Autodesk Inventor part; units mm, degrees
(part 11 of 13)
  arc A3938 (16.5247, 22.3668) -> (16.5247, 22.5192) centre (16.5247, 22.443) ccw
  line L3943 (16.5247, 22.5192) -> (15.4062, 22.5192)
  arc A3939 (15.4062, 22.5192) -> (15.4062, 22.3668) centre (15.4062, 22.443) ccw
  line L3944 (16.6009, 22.0702) -> (16.6009, 22.8159)
  arc A3940 (16.6009, 22.8159) -> (16.4485, 22.8159) centre (16.5247, 22.8159) ccw
  line L3945 (16.4485, 22.8159) -> (16.4485, 22.0702)
  arc A3941 (16.4485, 22.0702) -> (16.6009, 22.0702) centre (16.5247, 22.0702) ccw
  line L3946 (15.4824, 23.2395) -> (15.4824, 23.6123)
  arc A3942 (15.4824, 23.6123) -> (15.33, 23.6123) centre (15.4062, 23.6123) ccw
  line L3947 (15.33, 23.6123) -> (15.33, 23.2395)
  arc A3943 (15.33, 23.2395) -> (15.4824, 23.2395) centre (15.4062, 23.2395) ccw
  line L3948 (15.4062, 23.3497) -> (16.5247, 23.3497)
  arc A3944 (16.5247, 23.3497) -> (16.5247, 23.5021) centre (16.5247, 23.4259) ccw
  line L3949 (16.5247, 23.5021) -> (15.4062, 23.5021)
  arc A3945 (15.4062, 23.5021) -> (15.4062, 23.3497) centre (15.4062, 23.4259) ccw
  line L3950 (16.6009, 23.2395) -> (16.6009, 23.6123)
  arc A3946 (16.6009, 23.6123) -> (16.4485, 23.6123) centre (16.5247, 23.6123) ccw
  line L3951 (16.4485, 23.6123) -> (16.4485, 23.2395)
  arc A3947 (16.4485, 23.2395) -> (16.6009, 23.2395) centre (16.5247, 23.2395) ccw
  line L3952 (16.4485, 24.5782) -> (16.4485, 24.2054)
  arc A3948 (16.4485, 24.2054) -> (16.6009, 24.2054) centre (16.5247, 24.2054) ccw
  line L3953 (16.6009, 24.2054) -> (16.6009, 24.5782)
  arc A3949 (16.6009, 24.5782) -> (16.4485, 24.5782) centre (16.5247, 24.5782) ccw
  line L3954 (16.4708, 24.2593) -> (16.2844, 24.0729)
  arc A3950 (16.2844, 24.0729) -> (16.3922, 23.9651) centre (16.3383, 24.019) ccw
  line L3955 (16.3922, 23.9651) -> (16.5786, 24.1515)
  arc A3951 (16.5786, 24.1515) -> (16.4708, 24.2593) centre (16.5247, 24.2054) ccw
  line L3956 (16.3383, 24.0952) -> (15.5926, 24.0952)
  arc A3952 (15.5926, 24.0952) -> (15.5926, 23.9428) centre (15.5926, 24.019) ccw
  line L3957 (15.5926, 23.9428) -> (16.3383, 23.9428)
  arc A3953 (16.3383, 23.9428) -> (16.3383, 24.0952) centre (16.3383, 24.019) ccw
  line L3958 (15.6465, 24.0729) -> (15.4601, 24.2593)
  arc A3954 (15.4601, 24.2593) -> (15.3523, 24.1515) centre (15.4062, 24.2054) ccw
  line L3959 (15.3523, 24.1515) -> (15.5387, 23.9651)
  arc A3955 (15.5387, 23.9651) -> (15.6465, 24.0729) centre (15.5926, 24.019) ccw
  line L3960 (15.4824, 24.2054) -> (15.4824, 24.5782)
  arc A3956 (15.4824, 24.5782) -> (15.33, 24.5782) centre (15.4062, 24.5782) ccw
  line L3961 (15.33, 24.5782) -> (15.33, 24.2054)
  arc A3957 (15.33, 24.2054) -> (15.4824, 24.2054) centre (15.4062, 24.2054) ccw
  line L3962 (15.4601, 24.5243) -> (15.6465, 24.7108)
  arc A3958 (15.6465, 24.7108) -> (15.5387, 24.8186) centre (15.5926, 24.7647) ccw
  line L3963 (15.5387, 24.8186) -> (15.3523, 24.6321)
  arc A3959 (15.3523, 24.6321) -> (15.4601, 24.5243) centre (15.4062, 24.5782) ccw
  line L3964 (15.5926, 24.6885) -> (16.3383, 24.6885)
  arc A3960 (16.3383, 24.6885) -> (16.3383, 24.8409) centre (16.3383, 24.7647) ccw
  line L3965 (16.3383, 24.8409) -> (15.5926, 24.8409)
  arc A3961 (15.5926, 24.8409) -> (15.5926, 24.6885) centre (15.5926, 24.7647) ccw
  line L3966 (16.2844, 24.7108) -> (16.4708, 24.5243)
  arc A3962 (16.4708, 24.5243) -> (16.5786, 24.6321) centre (16.5247, 24.5782) ccw
  line L3967 (16.5786, 24.6321) -> (16.3922, 24.8186)
  arc A3963 (16.3922, 24.8186) -> (16.2844, 24.7108) centre (16.3383, 24.7647) ccw
  line L3968 (15.4062, 25.1121) -> (16.5247, 25.1121)
  arc A3964 (16.5247, 25.1121) -> (16.5247, 25.2645) centre (16.5247, 25.1883) ccw
  line L3969 (16.5247, 25.2645) -> (15.4062, 25.2645)
  arc A3965 (15.4062, 25.2645) -> (15.4062, 25.1121) centre (15.4062, 25.1883) ccw
  line L3970 (16.567, 25.2517) -> (15.4485, 25.9974)
  arc A3966 (15.4485, 25.9974) -> (15.3639, 25.8706) centre (15.4062, 25.934) ccw
  line L3971 (15.3639, 25.8706) -> (16.4824, 25.1249)
  arc A3967 (16.4824, 25.1249) -> (16.567, 25.2517) centre (16.5247, 25.1883) ccw
  line L3972 (15.4062, 25.8578) -> (16.5247, 25.8578)
  arc A3968 (16.5247, 25.8578) -> (16.5247, 26.0102) centre (16.5247, 25.934) ccw
  line L3973 (16.5247, 26.0102) -> (15.4062, 26.0102)
  arc A3969 (15.4062, 26.0102) -> (15.4062, 25.8578) centre (15.4062, 25.934) ccw
  line L3974 (15.4062, 27.4507) -> (16.5247, 27.4507)
  arc A3970 (16.5247, 27.4507) -> (16.5247, 27.6031) centre (16.5247, 27.5269) ccw
  line L3975 (16.5247, 27.6031) -> (15.4062, 27.6031)
  arc A3971 (15.4062, 27.6031) -> (15.4062, 27.4507) centre (15.4062, 27.5269) ccw
  line L3976 (16.6009, 27.5269) -> (16.6009, 28.0861)
  arc A3972 (16.6009, 28.0861) -> (16.4485, 28.0861) centre (16.5247, 28.0861) ccw
  line L3977 (16.4485, 28.0861) -> (16.4485, 27.5269)
  arc A3973 (16.4485, 27.5269) -> (16.6009, 27.5269) centre (16.5247, 27.5269) ccw
  line L3978 (16.5786, 28.14) -> (16.3922, 28.3265)
  arc A3974 (16.3922, 28.3265) -> (16.2844, 28.2187) centre (16.3383, 28.2726) ccw
  line L3979 (16.2844, 28.2187) -> (16.4708, 28.0322)
  arc A3975 (16.4708, 28.0322) -> (16.5786, 28.14) centre (16.5247, 28.0861) ccw
  line L3980 (16.3383, 28.3488) -> (16.1519, 28.3488)
  arc A3976 (16.1519, 28.3488) -> (16.1519, 28.1964) centre (16.1519, 28.2726) ccw
  line L3981 (16.1519, 28.1964) -> (16.3383, 28.1964)
  arc A3977 (16.3383, 28.1964) -> (16.3383, 28.3488) centre (16.3383, 28.2726) ccw
  line L3982 (16.098, 28.3265) -> (15.9115, 28.14)
  arc A3978 (15.9115, 28.14) -> (16.0193, 28.0322) centre (15.9654, 28.0861) ccw
  line L3983 (16.0193, 28.0322) -> (16.2058, 28.2187)
  arc A3979 (16.2058, 28.2187) -> (16.098, 28.3265) centre (16.1519, 28.2726) ccw
  line L3984 (16.0193, 28.14) -> (15.8329, 28.3265)
  arc A3980 (15.8329, 28.3265) -> (15.7251, 28.2187) centre (15.779, 28.2726) ccw
  line L3985 (15.7251, 28.2187) -> (15.9115, 28.0322)
  arc A3981 (15.9115, 28.0322) -> (16.0193, 28.14) centre (15.9654, 28.0861) ccw
  line L3986 (15.779, 28.3488) -> (15.5926, 28.3488)
  arc A3982 (15.5926, 28.3488) -> (15.5926, 28.1964) centre (15.5926, 28.2726) ccw
  line L3987 (15.5926, 28.1964) -> (15.779, 28.1964)
  arc A3983 (15.779, 28.1964) -> (15.779, 28.3488) centre (15.779, 28.2726) ccw
  line L3988 (15.5387, 28.3265) -> (15.3523, 28.14)
  arc A3984 (15.3523, 28.14) -> (15.4601, 28.0322) centre (15.4062, 28.0861) ccw
  line L3989 (15.4601, 28.0322) -> (15.6465, 28.2187)
  arc A3985 (15.6465, 28.2187) -> (15.5387, 28.3265) centre (15.5926, 28.2726) ccw
  line L3990 (15.33, 28.0861) -> (15.33, 27.5269)
  arc A3986 (15.33, 27.5269) -> (15.4824, 27.5269) centre (15.4062, 27.5269) ccw
  line L3991 (15.4824, 27.5269) -> (15.4824, 28.0861)
  arc A3987 (15.4824, 28.0861) -> (15.33, 28.0861) centre (15.4062, 28.0861) ccw
  line L3992 (16.0416, 27.5269) -> (16.0416, 28.0861)
  arc A3988 (16.0416, 28.0861) -> (15.8892, 28.0861) centre (15.9654, 28.0861) ccw
  line L3993 (15.8892, 28.0861) -> (15.8892, 27.5269)
  arc A3989 (15.8892, 27.5269) -> (16.0416, 27.5269) centre (15.9654, 27.5269) ccw
  line L3994 (16.4485, 29.2554) -> (16.4485, 28.8826)
  arc A3990 (16.4485, 28.8826) -> (16.6009, 28.8826) centre (16.5247, 28.8826) ccw
  line L3995 (16.6009, 28.8826) -> (16.6009, 29.2554)
  arc A3991 (16.6009, 29.2554) -> (16.4485, 29.2554) centre (16.5247, 29.2554) ccw
  line L3996 (16.4708, 28.9365) -> (16.2844, 28.7501)
  arc A3992 (16.2844, 28.7501) -> (16.3922, 28.6423) centre (16.3383, 28.6962) ccw
  line L3997 (16.3922, 28.6423) -> (16.5786, 28.8287)
  arc A3993 (16.5786, 28.8287) -> (16.4708, 28.9365) centre (16.5247, 28.8826) ccw
  line L3998 (16.3383, 28.7724) -> (15.5926, 28.7724)
  arc A3994 (15.5926, 28.7724) -> (15.5926, 28.62) centre (15.5926, 28.6962) ccw
  line L3999 (15.5926, 28.62) -> (16.3383, 28.62)
  arc A3995 (16.3383, 28.62) -> (16.3383, 28.7724) centre (16.3383, 28.6962) ccw
  line L4000 (15.6465, 28.7501) -> (15.4601, 28.9365)
  arc A3996 (15.4601, 28.9365) -> (15.3523, 28.8287) centre (15.4062, 28.8826) ccw
  line L4001 (15.3523, 28.8287) -> (15.5387, 28.6423)
  arc A3997 (15.5387, 28.6423) -> (15.6465, 28.7501) centre (15.5926, 28.6962) ccw
  line L4002 (15.4824, 28.8826) -> (15.4824, 29.2554)
  arc A3998 (15.4824, 29.2554) -> (15.33, 29.2554) centre (15.4062, 29.2554) ccw
  line L4003 (15.33, 29.2554) -> (15.33, 28.8826)
  arc A3999 (15.33, 28.8826) -> (15.4824, 28.8826) centre (15.4062, 28.8826) ccw
  line L4004 (15.4601, 29.2015) -> (15.6465, 29.388)
  arc A4000 (15.6465, 29.388) -> (15.5387, 29.4958) centre (15.5926, 29.4419) ccw
  line L4005 (15.5387, 29.4958) -> (15.3523, 29.3093)
  arc A4001 (15.3523, 29.3093) -> (15.4601, 29.2015) centre (15.4062, 29.2554) ccw
  line L4006 (15.5926, 29.3657) -> (16.3383, 29.3657)
  arc A4002 (16.3383, 29.3657) -> (16.3383, 29.5181) centre (16.3383, 29.4419) ccw
  line L4007 (16.3383, 29.5181) -> (15.5926, 29.5181)
  arc A4003 (15.5926, 29.5181) -> (15.5926, 29.3657) centre (15.5926, 29.4419) ccw
  line L4008 (16.2844, 29.388) -> (16.4708, 29.2015)
  arc A4004 (16.4708, 29.2015) -> (16.5786, 29.3093) centre (16.5247, 29.2554) ccw
  line L4009 (16.5786, 29.3093) -> (16.3922, 29.4958)
  arc A4005 (16.3922, 29.4958) -> (16.2844, 29.388) centre (16.3383, 29.4419) ccw
  line L4010 (15.4062, 29.7893) -> (16.1519, 29.7893)
  arc A4006 (16.1519, 29.7893) -> (16.1519, 29.9417) centre (16.1519, 29.8655) ccw
  line L4011 (16.1519, 29.9417) -> (15.4062, 29.9417)
  arc A4007 (15.4062, 29.9417) -> (15.4062, 29.7893) centre (15.4062, 29.8655) ccw
  line L4012 (16.2058, 29.8116) -> (16.5786, 30.1844)
  arc A4008 (16.5786, 30.1844) -> (16.4708, 30.2922) centre (16.5247, 30.2383) ccw
  line L4013 (16.4708, 30.2922) -> (16.098, 29.9194)
  arc A4009 (16.098, 29.9194) -> (16.2058, 29.8116) centre (16.1519, 29.8655) ccw
  line L4014 (16.5786, 30.2922) -> (16.2058, 30.6651)
  arc A4010 (16.2058, 30.6651) -> (16.098, 30.5573) centre (16.1519, 30.6112) ccw
  line L4015 (16.098, 30.5573) -> (16.4708, 30.1844)
  arc A4011 (16.4708, 30.1844) -> (16.5786, 30.2922) centre (16.5247, 30.2383) ccw
  line L4016 (16.1519, 30.6874) -> (15.4062, 30.6874)
  arc A4012 (15.4062, 30.6874) -> (15.4062, 30.535) centre (15.4062, 30.6112) ccw
  line L4017 (15.4062, 30.535) -> (16.1519, 30.535)
  arc A4013 (16.1519, 30.535) -> (16.1519, 30.6874) centre (16.1519, 30.6112) ccw
  line L4018 (16.0416, 29.8655) -> (16.0416, 30.6112)
  arc A4014 (16.0416, 30.6112) -> (15.8892, 30.6112) centre (15.9654, 30.6112) ccw
  line L4019 (15.8892, 30.6112) -> (15.8892, 29.8655)
  arc A4015 (15.8892, 29.8655) -> (16.0416, 29.8655) centre (15.9654, 29.8655) ccw
  line L4020 (15.4062, 30.9586) -> (16.5247, 30.9586)
  arc A4016 (16.5247, 30.9586) -> (16.5247, 31.111) centre (16.5247, 31.0348) ccw
  line L4021 (16.5247, 31.111) -> (15.4062, 31.111)
  arc A4017 (15.4062, 31.111) -> (15.4062, 30.9586) centre (15.4062, 31.0348) ccw
  line L4022 (16.6009, 31.0348) -> (16.6009, 31.594)
  arc A4018 (16.6009, 31.594) -> (16.4485, 31.594) centre (16.5247, 31.594) ccw
  line L4023 (16.4485, 31.594) -> (16.4485, 31.0348)
  arc A4019 (16.4485, 31.0348) -> (16.6009, 31.0348) centre (16.5247, 31.0348) ccw
  line L4024 (16.5786, 31.6479) -> (16.3922, 31.8344)
  arc A4020 (16.3922, 31.8344) -> (16.2844, 31.7266) centre (16.3383, 31.7805) ccw
  line L4025 (16.2844, 31.7266) -> (16.4708, 31.5401)
  arc A4021 (16.4708, 31.5401) -> (16.5786, 31.6479) centre (16.5247, 31.594) ccw
  line L4026 (16.3383, 31.8567) -> (15.9654, 31.8567)
  arc A4022 (15.9654, 31.8567) -> (15.9654, 31.7043) centre (15.9654, 31.7805) ccw
  line L4027 (15.9654, 31.7043) -> (16.3383, 31.7043)
  arc A4023 (16.3383, 31.7043) -> (16.3383, 31.8567) centre (16.3383, 31.7805) ccw
  line L4028 (15.9115, 31.8344) -> (15.7251, 31.6479)
  arc A4024 (15.7251, 31.6479) -> (15.8329, 31.5401) centre (15.779, 31.594) ccw
  line L4029 (15.8329, 31.5401) -> (16.0193, 31.7266)
  arc A4025 (16.0193, 31.7266) -> (15.9115, 31.8344) centre (15.9654, 31.7805) ccw
  line L4030 (15.7028, 31.594) -> (15.7028, 31.0348)
  arc A4026 (15.7028, 31.0348) -> (15.8552, 31.0348) centre (15.779, 31.0348) ccw
  line L4031 (15.8552, 31.0348) -> (15.8552, 31.594)
  arc A4027 (15.8552, 31.594) -> (15.7028, 31.594) centre (15.779, 31.594) ccw
  line L4032 (15.8329, 31.4615) -> (15.4601, 31.8344)
  arc A4028 (15.4601, 31.8344) -> (15.3523, 31.7266) centre (15.4062, 31.7805) ccw
  line L4033 (15.3523, 31.7266) -> (15.7251, 31.3537)
  arc A4029 (15.7251, 31.3537) -> (15.8329, 31.4615) centre (15.779, 31.4076) ccw
  line L4034 (16.5247, 32.2803) -> (15.4062, 32.2803)
  arc A4030 (15.4062, 32.2803) -> (15.4062, 32.1279) centre (15.4062, 32.2041) ccw
  line L4035 (15.4062, 32.1279) -> (16.5247, 32.1279)
  arc A4031 (16.5247, 32.1279) -> (16.5247, 32.2803) centre (16.5247, 32.2041) ccw
  line L4036 (15.4824, 32.2041) -> (15.4824, 32.7633)
  arc A4032 (15.4824, 32.7633) -> (15.33, 32.7633) centre (15.4062, 32.7633) ccw
  line L4037 (15.33, 32.7633) -> (15.33, 32.2041)
  arc A4033 (15.33, 32.2041) -> (15.4824, 32.2041) centre (15.4062, 32.2041) ccw
  line L4038 (15.4601, 32.7094) -> (15.6465, 32.8959)
  arc A4034 (15.6465, 32.8959) -> (15.5387, 33.0037) centre (15.5926, 32.9498) ccw
  line L4039 (15.5387, 33.0037) -> (15.3523, 32.8172)
  arc A4035 (15.3523, 32.8172) -> (15.4601, 32.7094) centre (15.4062, 32.7633) ccw
  line L4040 (15.5926, 32.8736) -> (16.3383, 32.8736)
  arc A4036 (16.3383, 32.8736) -> (16.3383, 33.026) centre (16.3383, 32.9498) ccw
  line L4041 (16.3383, 33.026) -> (15.5926, 33.026)
  arc A4037 (15.5926, 33.026) -> (15.5926, 32.8736) centre (15.5926, 32.9498) ccw
  line L4042 (16.2844, 32.8959) -> (16.4708, 32.7094)
  arc A4038 (16.4708, 32.7094) -> (16.5786, 32.8172) centre (16.5247, 32.7633) ccw
  line L4043 (16.5786, 32.8172) -> (16.3922, 33.0037)
  arc A4039 (16.3922, 33.0037) -> (16.2844, 32.8959) centre (16.3383, 32.9498) ccw
  line L4044 (16.4485, 32.7633) -> (16.4485, 32.2041)
  arc A4040 (16.4485, 32.2041) -> (16.6009, 32.2041) centre (16.5247, 32.2041) ccw
  line L4045 (16.6009, 32.2041) -> (16.6009, 32.7633)
  arc A4041 (16.6009, 32.7633) -> (16.4485, 32.7633) centre (16.5247, 32.7633) ccw
  line L4046 (11.3544, 2.168) -> (11.5408, 1.9815)
  arc A4042 (11.5408, 1.9815) -> (11.6486, 2.0893) centre (11.5947, 2.0354) ccw
  line L4047 (11.6486, 2.0893) -> (11.4622, 2.2758)
  arc A4043 (11.4622, 2.2758) -> (11.3544, 2.168) centre (11.4083, 2.2219) ccw
  line L4048 (11.5185, 2.0354) -> (11.5185, 1.6626)
  arc A4044 (11.5185, 1.6626) -> (11.6709, 1.6626) centre (11.5947, 1.6626) ccw
  line L4049 (11.6709, 1.6626) -> (11.6709, 2.0354)
  arc A4045 (11.6709, 2.0354) -> (11.5185, 2.0354) centre (11.5947, 2.0354) ccw
  line L4050 (11.5408, 1.7165) -> (11.3544, 1.5301)
  arc A4046 (11.3544, 1.5301) -> (11.4622, 1.4223) centre (11.4083, 1.4762) ccw
  line L4051 (11.4622, 1.4223) -> (11.6486, 1.6087)
  arc A4047 (11.6486, 1.6087) -> (11.5408, 1.7165) centre (11.5947, 1.6626) ccw
  line L4052 (11.4083, 1.5524) -> (11.2219, 1.5524)
  arc A4048 (11.2219, 1.5524) -> (11.2219, 1.4) centre (11.2219, 1.4762) ccw
  line L4053 (11.2219, 1.4) -> (11.4083, 1.4)
  arc A4049 (11.4083, 1.4) -> (11.4083, 1.5524) centre (11.4083, 1.4762) ccw
  line L4054 (11.2758, 1.5301) -> (11.0893, 1.7165)
  arc A4050 (11.0893, 1.7165) -> (10.9815, 1.6087) centre (11.0354, 1.6626) ccw
  line L4055 (10.9815, 1.6087) -> (11.168, 1.4223)
  arc A4051 (11.168, 1.4223) -> (11.2758, 1.5301) centre (11.2219, 1.4762) ccw
  line L4056 (11.1116, 1.6626) -> (11.1116, 2.0354)
  arc A4052 (11.1116, 2.0354) -> (10.9592, 2.0354) centre (11.0354, 2.0354) ccw
  line L4057 (10.9592, 2.0354) -> (10.9592, 1.6626)
  arc A4053 (10.9592, 1.6626) -> (11.1116, 1.6626) centre (11.0354, 1.6626) ccw
  line L4058 (11.0893, 2.0893) -> (10.9029, 2.2758)
  arc A4054 (10.9029, 2.2758) -> (10.7951, 2.168) centre (10.849, 2.2219) ccw
  line L4059 (10.7951, 2.168) -> (10.9815, 1.9815)
  arc A4055 (10.9815, 1.9815) -> (11.0893, 2.0893) centre (11.0354, 2.0354) ccw
  line L4060 (10.849, 2.2981) -> (10.6626, 2.2981)
  arc A4056 (10.6626, 2.2981) -> (10.6626, 2.1457) centre (10.6626, 2.2219) ccw
  line L4061 (10.6626, 2.1457) -> (10.849, 2.1457)
  arc A4057 (10.849, 2.1457) -> (10.849, 2.2981) centre (10.849, 2.2219) ccw
  line L4062 (10.6087, 2.2758) -> (10.4223, 2.0893)
  arc A4058 (10.4223, 2.0893) -> (10.5301, 1.9815) centre (10.4762, 2.0354) ccw
  line L4063 (10.5301, 1.9815) -> (10.7165, 2.168)
  arc A4059 (10.7165, 2.168) -> (10.6087, 2.2758) centre (10.6626, 2.2219) ccw
  line L4064 (10.4, 2.0354) -> (10.4, 1.6626)
  arc A4060 (10.4, 1.6626) -> (10.5524, 1.6626) centre (10.4762, 1.6626) ccw
  line L4065 (10.5524, 1.6626) -> (10.5524, 2.0354)
  arc A4061 (10.5524, 2.0354) -> (10.4, 2.0354) centre (10.4762, 2.0354) ccw
  line L4066 (10.4223, 1.6087) -> (10.6087, 1.4223)
  arc A4062 (10.6087, 1.4223) -> (10.7165, 1.5301) centre (10.6626, 1.4762) ccw
  line L4067 (10.7165, 1.5301) -> (10.5301, 1.7165)
  arc A4063 (10.5301, 1.7165) -> (10.4223, 1.6087) centre (10.4762, 1.6626) ccw
  line L4068 (11.5185, 3.3912) -> (11.5185, 2.6455)
  arc A4064 (11.5185, 2.6455) -> (11.6709, 2.6455) centre (11.5947, 2.6455) ccw
  line L4069 (11.6709, 2.6455) -> (11.6709, 3.3912)
  arc A4065 (11.6709, 3.3912) -> (11.5185, 3.3912) centre (11.5947, 3.3912) ccw
  line L4070 (11.5947, 2.7217) -> (10.4762, 2.7217)
  arc A4066 (10.4762, 2.7217) -> (10.4762, 2.5693) centre (10.4762, 2.6455) ccw
  line L4071 (10.4762, 2.5693) -> (11.5947, 2.5693)
  arc A4067 (11.5947, 2.5693) -> (11.5947, 2.7217) centre (11.5947, 2.6455) ccw
  line L4072 (10.5524, 2.6455) -> (10.5524, 3.3912)
  arc A4068 (10.5524, 3.3912) -> (10.4, 3.3912) centre (10.4762, 3.3912) ccw
  line L4073 (10.4, 3.3912) -> (10.4, 2.6455)
  arc A4069 (10.4, 2.6455) -> (10.5524, 2.6455) centre (10.4762, 2.6455) ccw
  line L4074 (11.1116, 2.6455) -> (11.1116, 3.0183)
  arc A4070 (11.1116, 3.0183) -> (10.9592, 3.0183) centre (11.0354, 3.0183) ccw
  line L4075 (10.9592, 3.0183) -> (10.9592, 2.6455)
  arc A4071 (10.9592, 2.6455) -> (11.1116, 2.6455) centre (11.0354, 2.6455) ccw
  line L4076 (10.4762, 3.7386) -> (11.5947, 3.7386)
  arc A4072 (11.5947, 3.7386) -> (11.5947, 3.891) centre (11.5947, 3.8148) ccw
  line L4077 (11.5947, 3.891) -> (10.4762, 3.891)
  arc A4073 (10.4762, 3.891) -> (10.4762, 3.7386) centre (10.4762, 3.8148) ccw
  line L4078 (11.637, 3.8782) -> (10.5185, 4.6239)
  arc A4074 (10.5185, 4.6239) -> (10.4339, 4.4971) centre (10.4762, 4.5605) ccw
  line L4079 (10.4339, 4.4971) -> (11.5524, 3.7514)
  arc A4075 (11.5524, 3.7514) -> (11.637, 3.8782) centre (11.5947, 3.8148) ccw
  line L4080 (10.4762, 4.4843) -> (11.5947, 4.4843)
  arc A4076 (11.5947, 4.4843) -> (11.5947, 4.6367) centre (11.5947, 4.5605) ccw
  line L4081 (11.5947, 4.6367) -> (10.4762, 4.6367)
  arc A4077 (10.4762, 4.6367) -> (10.4762, 4.4843) centre (10.4762, 4.5605) ccw
  line L4082 (11.5947, 5.0603) -> (10.4762, 5.0603)
  arc A4078 (10.4762, 5.0603) -> (10.4762, 4.9079) centre (10.4762, 4.9841) ccw
  line L4083 (10.4762, 4.9079) -> (11.5947, 4.9079)
  arc A4079 (11.5947, 4.9079) -> (11.5947, 5.0603) centre (11.5947, 4.9841) ccw
  line L4084 (10.9029, 4.9302) -> (11.6486, 5.6759)
  arc A4080 (11.6486, 5.6759) -> (11.5408, 5.7837) centre (11.5947, 5.7298) ccw
  line L4085 (11.5408, 5.7837) -> (10.7951, 5.038)
  arc A4081 (10.7951, 5.038) -> (10.9029, 4.9302) centre (10.849, 4.9841) ccw
  line L4086 (11.0893, 5.2244) -> (10.5301, 5.7837)
  arc A4082 (10.5301, 5.7837) -> (10.4223, 5.6759) centre (10.4762, 5.7298) ccw
  line L4087 (10.4223, 5.6759) -> (10.9815, 5.1166)
  arc A4083 (10.9815, 5.1166) -> (11.0893, 5.2244) centre (11.0354, 5.1705) ccw
  line L4088 (11.5185, 6.7126) -> (11.5185, 6.3398)
  arc A4084 (11.5185, 6.3398) -> (11.6709, 6.3398) centre (11.5947, 6.3398) ccw
  line L4089 (11.6709, 6.3398) -> (11.6709, 6.7126)
  arc A4085 (11.6709, 6.7126) -> (11.5185, 6.7126) centre (11.5947, 6.7126) ccw
  line L4090 (11.5408, 6.3937) -> (11.3544, 6.2073)
  arc A4086 (11.3544, 6.2073) -> (11.4622, 6.0995) centre (11.4083, 6.1534) ccw
  line L4091 (11.4622, 6.0995) -> (11.6486, 6.2859)
  arc A4087 (11.6486, 6.2859) -> (11.5408, 6.3937) centre (11.5947, 6.3398) ccw
  line L4092 (11.4083, 6.2296) -> (10.6626, 6.2296)
  arc A4088 (10.6626, 6.2296) -> (10.6626, 6.0772) centre (10.6626, 6.1534) ccw
  line L4093 (10.6626, 6.0772) -> (11.4083, 6.0772)
  arc A4089 (11.4083, 6.0772) -> (11.4083, 6.2296) centre (11.4083, 6.1534) ccw
  line L4094 (10.7165, 6.2073) -> (10.5301, 6.3937)
  arc A4090 (10.5301, 6.3937) -> (10.4223, 6.2859) centre (10.4762, 6.3398) ccw
  line L4095 (10.4223, 6.2859) -> (10.6087, 6.0995)
  arc A4091 (10.6087, 6.0995) -> (10.7165, 6.2073) centre (10.6626, 6.1534) ccw
  line L4096 (10.5524, 6.3398) -> (10.5524, 6.7126)
  arc A4092 (10.5524, 6.7126) -> (10.4, 6.7126) centre (10.4762, 6.7126) ccw
  line L4097 (10.4, 6.7126) -> (10.4, 6.3398)
  arc A4093 (10.4, 6.3398) -> (10.5524, 6.3398) centre (10.4762, 6.3398) ccw
  line L4098 (10.5301, 6.6587) -> (10.7165, 6.8452)
  arc A4094 (10.7165, 6.8452) -> (10.6087, 6.953) centre (10.6626, 6.8991) ccw
  line L4099 (10.6087, 6.953) -> (10.4223, 6.7665)
  arc A4095 (10.4223, 6.7665) -> (10.5301, 6.6587) centre (10.4762, 6.7126) ccw
  line L4100 (10.6626, 6.8229) -> (11.4083, 6.8229)
  arc A4096 (11.4083, 6.8229) -> (11.4083, 6.9753) centre (11.4083, 6.8991) ccw
  line L4101 (11.4083, 6.9753) -> (10.6626, 6.9753)
  arc A4097 (10.6626, 6.9753) -> (10.6626, 6.8229) centre (10.6626, 6.8991) ccw
  line L4102 (11.3544, 6.8452) -> (11.5408, 6.6587)
  arc A4098 (11.5408, 6.6587) -> (11.6486, 6.7665) centre (11.5947, 6.7126) ccw
  line L4103 (11.6486, 6.7665) -> (11.4622, 6.953)
  arc A4099 (11.4622, 6.953) -> (11.3544, 6.8452) centre (11.4083, 6.8991) ccw
  line L4104 (11.5947, 8.5682) -> (10.4762, 8.5682)
  arc A4100 (10.4762, 8.5682) -> (10.4762, 8.4158) centre (10.4762, 8.492) ccw
  line L4105 (10.4762, 8.4158) -> (11.5947, 8.4158)
  arc A4101 (11.5947, 8.4158) -> (11.5947, 8.5682) centre (11.5947, 8.492) ccw
  line L4106 (10.5524, 8.492) -> (10.5524, 9.2377)
  arc A4102 (10.5524, 9.2377) -> (10.4, 9.2377) centre (10.4762, 9.2377) ccw
  line L4107 (10.4, 9.2377) -> (10.4, 8.492)
  arc A4103 (10.4, 8.492) -> (10.5524, 8.492) centre (10.4762, 8.492) ccw
  line L4108 (10.4762, 9.5851) -> (11.2219, 9.5851)
  arc A4104 (11.2219, 9.5851) -> (11.2219, 9.7375) centre (11.2219, 9.6613) ccw
  line L4109 (11.2219, 9.7375) -> (10.4762, 9.7375)
  arc A4105 (10.4762, 9.7375) -> (10.4762, 9.5851) centre (10.4762, 9.6613) ccw
  line L4110 (11.2758, 9.6074) -> (11.6486, 9.9802)
  arc A4106 (11.6486, 9.9802) -> (11.5408, 10.088) centre (11.5947, 10.0341) ccw
  line L4111 (11.5408, 10.088) -> (11.168, 9.7152)
  arc A4107 (11.168, 9.7152) -> (11.2758, 9.6074) centre (11.2219, 9.6613) ccw
  line L4112 (11.6486, 10.088) -> (11.2758, 10.4609)
  arc A4108 (11.2758, 10.4609) -> (11.168, 10.3531) centre (11.2219, 10.407) ccw
  line L4113 (11.168, 10.3531) -> (11.5408, 9.9802)
  arc A4109 (11.5408, 9.9802) -> (11.6486, 10.088) centre (11.5947, 10.0341) ccw
  line L4114 (11.2219, 10.4832) -> (10.4762, 10.4832)
  arc A4110 (10.4762, 10.4832) -> (10.4762, 10.3308) centre (10.4762, 10.407) ccw
  line L4115 (10.4762, 10.3308) -> (11.2219, 10.3308)
  arc A4111 (11.2219, 10.3308) -> (11.2219, 10.4832) centre (11.2219, 10.407) ccw
  line L4116 (11.1116, 9.6613) -> (11.1116, 10.407)
  arc A4112 (11.1116, 10.407) -> (10.9592, 10.407) centre (11.0354, 10.407) ccw
  line L4117 (10.9592, 10.407) -> (10.9592, 9.6613)
  arc A4113 (10.9592, 9.6613) -> (11.1116, 9.6613) centre (11.0354, 9.6613) ccw
  line L4118 (10.4762, 10.7544) -> (11.5947, 10.7544)
  arc A4114 (11.5947, 10.7544) -> (11.5947, 10.9068) centre (11.5947, 10.8306) ccw
  line L4119 (11.5947, 10.9068) -> (10.4762, 10.9068)
  arc A4115 (10.4762, 10.9068) -> (10.4762, 10.7544) centre (10.4762, 10.8306) ccw
  line L4120 (11.6709, 10.8306) -> (11.6709, 11.3898)
  arc A4116 (11.6709, 11.3898) -> (11.5185, 11.3898) centre (11.5947, 11.3898) ccw
  line L4121 (11.5185, 11.3898) -> (11.5185, 10.8306)
  arc A4117 (11.5185, 10.8306) -> (11.6709, 10.8306) centre (11.5947, 10.8306) ccw
  line L4122 (11.6486, 11.4437) -> (11.4622, 11.6302)
  arc A4118 (11.4622, 11.6302) -> (11.3544, 11.5224) centre (11.4083, 11.5763) ccw
  line L4123 (11.3544, 11.5224) -> (11.5408, 11.3359)
  arc A4119 (11.5408, 11.3359) -> (11.6486, 11.4437) centre (11.5947, 11.3898) ccw
  line L4124 (11.4083, 11.6525) -> (11.2219, 11.6525)
  arc A4120 (11.2219, 11.6525) -> (11.2219, 11.5001) centre (11.2219, 11.5763) ccw
  line L4125 (11.2219, 11.5001) -> (11.4083, 11.5001)
  arc A4121 (11.4083, 11.5001) -> (11.4083, 11.6525) centre (11.4083, 11.5763) ccw
  line L4126 (11.168, 11.6302) -> (10.9815, 11.4437)
  arc A4122 (10.9815, 11.4437) -> (11.0893, 11.3359) centre (11.0354, 11.3898) ccw
  line L4127 (11.0893, 11.3359) -> (11.2758, 11.5224)
  arc A4123 (11.2758, 11.5224) -> (11.168, 11.6302) centre (11.2219, 11.5763) ccw
  line L4128 (11.0893, 11.4437) -> (10.9029, 11.6302)
  arc A4124 (10.9029, 11.6302) -> (10.7951, 11.5224) centre (10.849, 11.5763) ccw
  line L4129 (10.7951, 11.5224) -> (10.9815, 11.3359)
  arc A4125 (10.9815, 11.3359) -> (11.0893, 11.4437) centre (11.0354, 11.3898) ccw
  line L4130 (10.849, 11.6525) -> (10.6626, 11.6525)
  arc A4126 (10.6626, 11.6525) -> (10.6626, 11.5001) centre (10.6626, 11.5763) ccw
  line L4131 (10.6626, 11.5001) -> (10.849, 11.5001)
  arc A4127 (10.849, 11.5001) -> (10.849, 11.6525) centre (10.849, 11.5763) ccw
  line L4132 (10.6087, 11.6302) -> (10.4223, 11.4437)
  arc A4128 (10.4223, 11.4437) -> (10.5301, 11.3359) centre (10.4762, 11.3898) ccw
  line L4133 (10.5301, 11.3359) -> (10.7165, 11.5224)
  arc A4129 (10.7165, 11.5224) -> (10.6087, 11.6302) centre (10.6626, 11.5763) ccw
  line L4134 (10.4, 11.3898) -> (10.4, 10.8306)
  arc A4130 (10.4, 10.8306) -> (10.5524, 10.8306) centre (10.4762, 10.8306) ccw
  line L4135 (10.5524, 10.8306) -> (10.5524, 11.3898)
  arc A4131 (10.5524, 11.3898) -> (10.4, 11.3898) centre (10.4762, 11.3898) ccw
  line L4136 (11.1116, 10.8306) -> (11.1116, 11.3898)
  arc A4132 (11.1116, 11.3898) -> (10.9592, 11.3898) centre (11.0354, 11.3898) ccw
  line L4137 (10.9592, 11.3898) -> (10.9592, 10.8306)
  arc A4133 (10.9592, 10.8306) -> (11.1116, 10.8306) centre (11.0354, 10.8306) ccw
  line L4138 (10.4762, 13.093) -> (11.5947, 13.093)
  arc A4134 (11.5947, 13.093) -> (11.5947, 13.2454) centre (11.5947, 13.1692) ccw
  line L4139 (11.5947, 13.2454) -> (10.4762, 13.2454)
  arc A4135 (10.4762, 13.2454) -> (10.4762, 13.093) centre (10.4762, 13.1692) ccw
  line L4140 (11.6709, 13.1692) -> (11.6709, 13.7284)
  arc A4136 (11.6709, 13.7284) -> (11.5185, 13.7284) centre (11.5947, 13.7284) ccw
  line L4141 (11.5185, 13.7284) -> (11.5185, 13.1692)
  arc A4137 (11.5185, 13.1692) -> (11.6709, 13.1692) centre (11.5947, 13.1692) ccw
  line L4142 (11.6486, 13.7823) -> (11.4622, 13.9688)
  arc A4138 (11.4622, 13.9688) -> (11.3544, 13.861) centre (11.4083, 13.9149) ccw
  line L4143 (11.3544, 13.861) -> (11.5408, 13.6745)
  arc A4139 (11.5408, 13.6745) -> (11.6486, 13.7823) centre (11.5947, 13.7284) ccw
  line L4144 (11.4083, 13.9911) -> (11.0354, 13.9911)
  arc A4140 (11.0354, 13.9911) -> (11.0354, 13.8387) centre (11.0354, 13.9149) ccw
  line L4145 (11.0354, 13.8387) -> (11.4083, 13.8387)
  arc A4141 (11.4083, 13.8387) -> (11.4083, 13.9911) centre (11.4083, 13.9149) ccw
  line L4146 (10.9815, 13.9688) -> (10.7951, 13.7823)
  arc A4142 (10.7951, 13.7823) -> (10.9029, 13.6745) centre (10.849, 13.7284) ccw
  line L4147 (10.9029, 13.6745) -> (11.0893, 13.861)
  arc A4143 (11.0893, 13.861) -> (10.9815, 13.9688) centre (11.0354, 13.9149) ccw
  line L4148 (10.7728, 13.7284) -> (10.7728, 13.1692)
  arc A4144 (10.7728, 13.1692) -> (10.9252, 13.1692) centre (10.849, 13.1692) ccw
  line L4149 (10.9252, 13.1692) -> (10.9252, 13.7284)
  arc A4145 (10.9252, 13.7284) -> (10.7728, 13.7284) centre (10.849, 13.7284) ccw
  line L4150 (11.5185, 14.8977) -> (11.5185, 14.5249)
  arc A4146 (11.5185, 14.5249) -> (11.6709, 14.5249) centre (11.5947, 14.5249) ccw
  line L4151 (11.6709, 14.5249) -> (11.6709, 14.8977)
  arc A4147 (11.6709, 14.8977) -> (11.5185, 14.8977) centre (11.5947, 14.8977) ccw
  line L4152 (11.5408, 14.5788) -> (11.3544, 14.3924)
  arc A4148 (11.3544, 14.3924) -> (11.4622, 14.2846) centre (11.4083, 14.3385) ccw
  line L4153 (11.4622, 14.2846) -> (11.6486, 14.471)
  arc A4149 (11.6486, 14.471) -> (11.5408, 14.5788) centre (11.5947, 14.5249) ccw
  line L4154 (11.4083, 14.4147) -> (10.6626, 14.4147)
  arc A4150 (10.6626, 14.4147) -> (10.6626, 14.2623) centre (10.6626, 14.3385) ccw
  line L4155 (10.6626, 14.2623) -> (11.4083, 14.2623)
  arc A4151 (11.4083, 14.2623) -> (11.4083, 14.4147) centre (11.4083, 14.3385) ccw
  line L4156 (10.7165, 14.3924) -> (10.5301, 14.5788)
  arc A4152 (10.5301, 14.5788) -> (10.4223, 14.471) centre (10.4762, 14.5249) ccw
  line L4157 (10.4223, 14.471) -> (10.6087, 14.2846)
  arc A4153 (10.6087, 14.2846) -> (10.7165, 14.3924) centre (10.6626, 14.3385) ccw
  line L4158 (10.5524, 14.5249) -> (10.5524, 14.8977)
  arc A4154 (10.5524, 14.8977) -> (10.4, 14.8977) centre (10.4762, 14.8977) ccw
  line L4159 (10.4, 14.8977) -> (10.4, 14.5249)
  arc A4155 (10.4, 14.5249) -> (10.5524, 14.5249) centre (10.4762, 14.5249) ccw
  line L4160 (10.5301, 14.8438) -> (10.7165, 15.0303)
  arc A4156 (10.7165, 15.0303) -> (10.6087, 15.1381) centre (10.6626, 15.0842) ccw
  line L4161 (10.6087, 15.1381) -> (10.4223, 14.9516)
  arc A4157 (10.4223, 14.9516) -> (10.5301, 14.8438) centre (10.4762, 14.8977) ccw
  line L4162 (10.6626, 15.008) -> (11.4083, 15.008)
  arc A4158 (11.4083, 15.008) -> (11.4083, 15.1604) centre (11.4083, 15.0842) ccw
  line L4163 (11.4083, 15.1604) -> (10.6626, 15.1604)
  arc A4159 (10.6626, 15.1604) -> (10.6626, 15.008) centre (10.6626, 15.0842) ccw
  line L4164 (11.3544, 15.0303) -> (11.5408, 14.8438)
  arc A4160 (11.5408, 14.8438) -> (11.6486, 14.9516) centre (11.5947, 14.8977) ccw
  line L4165 (11.6486, 14.9516) -> (11.4622, 15.1381)
  arc A4161 (11.4622, 15.1381) -> (11.3544, 15.0303) centre (11.4083, 15.0842) ccw
  line L4166 (11.5947, 15.584) -> (10.4762, 15.584)
  arc A4162 (10.4762, 15.584) -> (10.4762, 15.4316) centre (10.4762, 15.5078) ccw
  line L4167 (10.4762, 15.4316) -> (11.5947, 15.4316)
  arc A4163 (11.5947, 15.4316) -> (11.5947, 15.584) centre (11.5947, 15.5078) ccw
  line L4168 (10.5301, 15.4539) -> (10.9029, 15.8267)
  arc A4164 (10.9029, 15.8267) -> (10.7951, 15.9345) centre (10.849, 15.8806) ccw
  line L4169 (10.7951, 15.9345) -> (10.4223, 15.5617)
  arc A4165 (10.4223, 15.5617) -> (10.5301, 15.4539) centre (10.4762, 15.5078) ccw
  line L4170 (10.9029, 15.9345) -> (10.5301, 16.3074)
  arc A4166 (10.5301, 16.3074) -> (10.4223, 16.1996) centre (10.4762, 16.2535) ccw
  line L4171 (10.4223, 16.1996) -> (10.7951, 15.8267)
  arc A4167 (10.7951, 15.8267) -> (10.9029, 15.9345) centre (10.849, 15.8806) ccw
  line L4172 (10.4762, 16.1773) -> (11.5947, 16.1773)
  arc A4168 (11.5947, 16.1773) -> (11.5947, 16.3297) centre (11.5947, 16.2535) ccw
  line L4173 (11.5947, 16.3297) -> (10.4762, 16.3297)
  arc A4169 (10.4762, 16.3297) -> (10.4762, 16.1773) centre (10.4762, 16.2535) ccw
  line L4174 (11.5185, 17.4228) -> (11.5185, 16.6771)
  arc A4170 (11.5185, 16.6771) -> (11.6709, 16.6771) centre (11.5947, 16.6771) ccw
  line L4175 (11.6709, 16.6771) -> (11.6709, 17.4228)
  arc A4171 (11.6709, 17.4228) -> (11.5185, 17.4228) centre (11.5947, 17.4228) ccw
  line L4176 (11.5947, 16.7533) -> (10.4762, 16.7533)
  arc A4172 (10.4762, 16.7533) -> (10.4762, 16.6009) centre (10.4762, 16.6771) ccw
  line L4177 (10.4762, 16.6009) -> (11.5947, 16.6009)
  arc A4173 (11.5947, 16.6009) -> (11.5947, 16.7533) centre (11.5947, 16.6771) ccw
  line L4178 (10.5524, 16.6771) -> (10.5524, 17.4228)
  arc A4174 (10.5524, 17.4228) -> (10.4, 17.4228) centre (10.4762, 17.4228) ccw
  line L4179 (10.4, 17.4228) -> (10.4, 16.6771)
  arc A4175 (10.4, 16.6771) -> (10.5524, 16.6771) centre (10.4762, 16.6771) ccw
  line L4180 (11.1116, 16.6771) -> (11.1116, 17.0499)
  arc A4176 (11.1116, 17.0499) -> (10.9592, 17.0499) centre (11.0354, 17.0499) ccw
  line L4181 (10.9592, 17.0499) -> (10.9592, 16.6771)
  arc A4177 (10.9592, 16.6771) -> (11.1116, 16.6771) centre (11.0354, 16.6771) ccw
  line L4182 (10.4762, 17.7702) -> (11.5947, 17.7702)
  arc A4178 (11.5947, 17.7702) -> (11.5947, 17.9226) centre (11.5947, 17.8464) ccw
  line L4183 (11.5947, 17.9226) -> (10.4762, 17.9226)
  arc A4179 (10.4762, 17.9226) -> (10.4762, 17.7702) centre (10.4762, 17.8464) ccw
  line L4184 (11.6709, 17.8464) -> (11.6709, 18.4056)
  arc A4180 (11.6709, 18.4056) -> (11.5185, 18.4056) centre (11.5947, 18.4056) ccw
  line L4185 (11.5185, 18.4056) -> (11.5185, 17.8464)
  arc A4181 (11.5185, 17.8464) -> (11.6709, 17.8464) centre (11.5947, 17.8464) ccw
  line L4186 (11.6486, 18.4595) -> (11.4622, 18.646)
  arc A4182 (11.4622, 18.646) -> (11.3544, 18.5382) centre (11.4083, 18.5921) ccw
  line L4187 (11.3544, 18.5382) -> (11.5408, 18.3517)
  arc A4183 (11.5408, 18.3517) -> (11.6486, 18.4595) centre (11.5947, 18.4056) ccw
  line L4188 (11.4083, 18.6683) -> (11.0354, 18.6683)
  arc A4184 (11.0354, 18.6683) -> (11.0354, 18.5159) centre (11.0354, 18.5921) ccw
  line L4189 (11.0354, 18.5159) -> (11.4083, 18.5159)
  arc A4185 (11.4083, 18.5159) -> (11.4083, 18.6683) centre (11.4083, 18.5921) ccw
  line L4190 (10.9815, 18.646) -> (10.7951, 18.4595)
  arc A4186 (10.7951, 18.4595) -> (10.9029, 18.3517) centre (10.849, 18.4056) ccw
  line L4191 (10.9029, 18.3517) -> (11.0893, 18.5382)
  arc A4187 (11.0893, 18.5382) -> (10.9815, 18.646) centre (11.0354, 18.5921) ccw
  line L4192 (10.7728, 18.4056) -> (10.7728, 17.8464)
  arc A4188 (10.7728, 17.8464) -> (10.9252, 17.8464) centre (10.849, 17.8464) ccw
  line L4193 (10.9252, 17.8464) -> (10.9252, 18.4056)
  arc A4189 (10.9252, 18.4056) -> (10.7728, 18.4056) centre (10.849, 18.4056) ccw
  line L4194 (10.9029, 18.2731) -> (10.5301, 18.646)
  arc A4190 (10.5301, 18.646) -> (10.4223, 18.5382) centre (10.4762, 18.5921) ccw
  line L4195 (10.4223, 18.5382) -> (10.7951, 18.1653)
  arc A4191 (10.7951, 18.1653) -> (10.9029, 18.2731) centre (10.849, 18.2192) ccw
  line L4196 (11.5947, 20.2612) -> (10.4762, 20.2612)
  arc A4192 (10.4762, 20.2612) -> (10.4762, 20.1088) centre (10.4762, 20.185) ccw
  line L4197 (10.4762, 20.1088) -> (11.5947, 20.1088)
  arc A4193 (11.5947, 20.1088) -> (11.5947, 20.2612) centre (11.5947, 20.185) ccw
  line L4198 (10.5524, 20.185) -> (10.5524, 20.7442)
  arc A4194 (10.5524, 20.7442) -> (10.4, 20.7442) centre (10.4762, 20.7442) ccw
  line L4199 (10.4, 20.7442) -> (10.4, 20.185)
  arc A4195 (10.4, 20.185) -> (10.5524, 20.185) centre (10.4762, 20.185) ccw
  line L4200 (10.5301, 20.6903) -> (10.7165, 20.8768)
  arc A4196 (10.7165, 20.8768) -> (10.6087, 20.9846) centre (10.6626, 20.9307) ccw
  line L4201 (10.6087, 20.9846) -> (10.4223, 20.7981)
  arc A4197 (10.4223, 20.7981) -> (10.5301, 20.6903) centre (10.4762, 20.7442) ccw
  line L4202 (10.6626, 20.8545) -> (11.4083, 20.8545)
  arc A4198 (11.4083, 20.8545) -> (11.4083, 21.0069) centre (11.4083, 20.9307) ccw
  line L4203 (11.4083, 21.0069) -> (10.6626, 21.0069)
  arc A4199 (10.6626, 21.0069) -> (10.6626, 20.8545) centre (10.6626, 20.9307) ccw
  line L4204 (11.3544, 20.8768) -> (11.5408, 20.6903)
  arc A4200 (11.5408, 20.6903) -> (11.6486, 20.7981) centre (11.5947, 20.7442) ccw
  line L4205 (11.6486, 20.7981) -> (11.4622, 20.9846)
  arc A4201 (11.4622, 20.9846) -> (11.3544, 20.8768) centre (11.4083, 20.9307) ccw
  line L4206 (11.5185, 20.7442) -> (11.5185, 20.185)
  arc A4202 (11.5185, 20.185) -> (11.6709, 20.185) centre (11.5947, 20.185) ccw
  line L4207 (11.6709, 20.185) -> (11.6709, 20.7442)
  arc A4203 (11.6709, 20.7442) -> (11.5185, 20.7442) centre (11.5947, 20.7442) ccw
  line L4208 (10.5524, 21.3543) -> (10.5524, 21.7271)
  arc A4204 (10.5524, 21.7271) -> (10.4, 21.7271) centre (10.4762, 21.7271) ccw
  line L4209 (10.4, 21.7271) -> (10.4, 21.3543)
  arc A4205 (10.4, 21.3543) -> (10.5524, 21.3543) centre (10.4762, 21.3543) ccw
  line L4210 (10.4762, 21.4645) -> (11.5947, 21.4645)
  arc A4206 (11.5947, 21.4645) -> (11.5947, 21.6169) centre (11.5947, 21.5407) ccw
  line L4211 (11.5947, 21.6169) -> (10.4762, 21.6169)
  arc A4207 (10.4762, 21.6169) -> (10.4762, 21.4645) centre (10.4762, 21.5407) ccw
  line L4212 (11.6709, 21.3543) -> (11.6709, 21.7271)
  arc A4208 (11.6709, 21.7271) -> (11.5185, 21.7271) centre (11.5947, 21.7271) ccw
  line L4213 (11.5185, 21.7271) -> (11.5185, 21.3543)
  arc A4209 (11.5185, 21.3543) -> (11.6709, 21.3543) centre (11.5947, 21.3543) ccw
  line L4214 (11.3544, 22.8256) -> (11.5408, 22.6391)
  arc A4210 (11.5408, 22.6391) -> (11.6486, 22.7469) centre (11.5947, 22.693) ccw
  line L4215 (11.6486, 22.7469) -> (11.4622, 22.9334)
  arc A4211 (11.4622, 22.9334) -> (11.3544, 22.8256) centre (11.4083, 22.8795) ccw
  line L4216 (11.5185, 22.693) -> (11.5185, 22.3202)
  arc A4212 (11.5185, 22.3202) -> (11.6709, 22.3202) centre (11.5947, 22.3202) ccw
  line L4217 (11.6709, 22.3202) -> (11.6709, 22.693)
  arc A4213 (11.6709, 22.693) -> (11.5185, 22.693) centre (11.5947, 22.693) ccw
  line L4218 (11.5408, 22.3741) -> (11.3544, 22.1877)
  arc A4214 (11.3544, 22.1877) -> (11.4622, 22.0799) centre (11.4083, 22.1338) ccw
  line L4219 (11.4622, 22.0799) -> (11.6486, 22.2663)
  arc A4215 (11.6486, 22.2663) -> (11.5408, 22.3741) centre (11.5947, 22.3202) ccw
  line L4220 (11.4083, 22.21) -> (11.2219, 22.21)
  arc A4216 (11.2219, 22.21) -> (11.2219, 22.0576) centre (11.2219, 22.1338) ccw
  line L4221 (11.2219, 22.0576) -> (11.4083, 22.0576)
  arc A4217 (11.4083, 22.0576) -> (11.4083, 22.21) centre (11.4083, 22.1338) ccw
  line L4222 (11.2758, 22.1877) -> (11.0893, 22.3741)
  arc A4218 (11.0893, 22.3741) -> (10.9815, 22.2663) centre (11.0354, 22.3202) ccw
  line L4223 (10.9815, 22.2663) -> (11.168, 22.0799)
  arc A4219 (11.168, 22.0799) -> (11.2758, 22.1877) centre (11.2219, 22.1338) ccw
  line L4224 (11.1116, 22.3202) -> (11.1116, 22.693)
  arc A4220 (11.1116, 22.693) -> (10.9592, 22.693) centre (11.0354, 22.693) ccw
  line L4225 (10.9592, 22.693) -> (10.9592, 22.3202)
  arc A4221 (10.9592, 22.3202) -> (11.1116, 22.3202) centre (11.0354, 22.3202) ccw
  line L4226 (11.0893, 22.7469) -> (10.9029, 22.9334)
  arc A4222 (10.9029, 22.9334) -> (10.7951, 22.8256) centre (10.849, 22.8795) ccw
  line L4227 (10.7951, 22.8256) -> (10.9815, 22.6391)
  arc A4223 (10.9815, 22.6391) -> (11.0893, 22.7469) centre (11.0354, 22.693) ccw
  line L4228 (10.849, 22.9557) -> (10.6626, 22.9557)
  arc A4224 (10.6626, 22.9557) -> (10.6626, 22.8033) centre (10.6626, 22.8795) ccw
  line L4229 (10.6626, 22.8033) -> (10.849, 22.8033)
  arc A4225 (10.849, 22.8033) -> (10.849, 22.9557) centre (10.849, 22.8795) ccw
  line L4230 (10.6087, 22.9334) -> (10.4223, 22.7469)
  arc A4226 (10.4223, 22.7469) -> (10.5301, 22.6391) centre (10.4762, 22.693) ccw
  line L4231 (10.5301, 22.6391) -> (10.7165, 22.8256)
  arc A4227 (10.7165, 22.8256) -> (10.6087, 22.9334) centre (10.6626, 22.8795) ccw
  line L4232 (10.4, 22.693) -> (10.4, 22.3202)
  arc A4228 (10.4, 22.3202) -> (10.5524, 22.3202) centre (10.4762, 22.3202) ccw
  line L4233 (10.5524, 22.3202) -> (10.5524, 22.693)
  arc A4229 (10.5524, 22.693) -> (10.4, 22.693) centre (10.4762, 22.693) ccw
  line L4234 (10.4223, 22.2663) -> (10.6087, 22.0799)
  arc A4230 (10.6087, 22.0799) -> (10.7165, 22.1877) centre (10.6626, 22.1338) ccw
  line L4235 (10.7165, 22.1877) -> (10.5301, 22.3741)
  arc A4231 (10.5301, 22.3741) -> (10.4223, 22.2663) centre (10.4762, 22.3202) ccw
  line L4236 (10.4762, 23.5997) -> (11.5947, 23.5997)
  arc A4232 (11.5947, 23.5997) -> (11.5947, 23.7521) centre (11.5947, 23.6759) ccw
  line L4237 (11.5947, 23.7521) -> (10.4762, 23.7521)
  arc A4233 (10.4762, 23.7521) -> (10.4762, 23.5997) centre (10.4762, 23.6759) ccw
  line L4238 (11.6709, 23.3031) -> (11.6709, 24.0488)
  arc A4234 (11.6709, 24.0488) -> (11.5185, 24.0488) centre (11.5947, 24.0488) ccw
  line L4239 (11.5185, 24.0488) -> (11.5185, 23.3031)
  arc A4235 (11.5185, 23.3031) -> (11.6709, 23.3031) centre (11.5947, 23.3031) ccw
  line L4240 (10.4762, 24.3962) -> (11.5947, 24.3962)
  arc A4236 (11.5947, 24.3962) -> (11.5947, 24.5486) centre (11.5947, 24.4724) ccw
  line L4241 (11.5947, 24.5486) -> (10.4762, 24.5486)
  arc A4237 (10.4762, 24.5486) -> (10.4762, 24.3962) centre (10.4762, 24.4724) ccw
  line L4242 (11.6709, 24.4724) -> (11.6709, 25.0316)
  arc A4238 (11.6709, 25.0316) -> (11.5185, 25.0316) centre (11.5947, 25.0316) ccw
  line L4243 (11.5185, 25.0316) -> (11.5185, 24.4724)
  arc A4239 (11.5185, 24.4724) -> (11.6709, 24.4724) centre (11.5947, 24.4724) ccw
  line L4244 (11.6486, 25.0855) -> (11.4622, 25.272)
  arc A4240 (11.4622, 25.272) -> (11.3544, 25.1642) centre (11.4083, 25.2181) ccw
  line L4245 (11.3544, 25.1642) -> (11.5408, 24.9777)
  arc A4241 (11.5408, 24.9777) -> (11.6486, 25.0855) centre (11.5947, 25.0316) ccw
  line L4246 (11.4083, 25.2943) -> (11.0354, 25.2943)
  arc A4242 (11.0354, 25.2943) -> (11.0354, 25.1419) centre (11.0354, 25.2181) ccw
  line L4247 (11.0354, 25.1419) -> (11.4083, 25.1419)
  arc A4243 (11.4083, 25.1419) -> (11.4083, 25.2943) centre (11.4083, 25.2181) ccw
  line L4248 (10.9815, 25.272) -> (10.7951, 25.0855)
  arc A4244 (10.7951, 25.0855) -> (10.9029, 24.9777) centre (10.849, 25.0316) ccw
  line L4249 (10.9029, 24.9777) -> (11.0893, 25.1642)
  arc A4245 (11.0893, 25.1642) -> (10.9815, 25.272) centre (11.0354, 25.2181) ccw
  line L4250 (10.7728, 25.0316) -> (10.7728, 24.4724)
  arc A4246 (10.7728, 24.4724) -> (10.9252, 24.4724) centre (10.849, 24.4724) ccw
  line L4251 (10.9252, 24.4724) -> (10.9252, 25.0316)
  arc A4247 (10.9252, 25.0316) -> (10.7728, 25.0316) centre (10.849, 25.0316) ccw
  line L4252 (10.9029, 24.8991) -> (10.5301, 25.272)
  arc A4248 (10.5301, 25.272) -> (10.4223, 25.1642) centre (10.4762, 25.2181) ccw
  line L4253 (10.4223, 25.1642) -> (10.7951, 24.7913)
  arc A4249 (10.7951, 24.7913) -> (10.9029, 24.8991) centre (10.849, 24.8452) ccw
  line L4254 (11.5185, 26.2009) -> (11.5185, 25.8281)
  arc A4250 (11.5185, 25.8281) -> (11.6709, 25.8281) centre (11.5947, 25.8281) ccw
  line L4255 (11.6709, 25.8281) -> (11.6709, 26.2009)
  arc A4251 (11.6709, 26.2009) -> (11.5185, 26.2009) centre (11.5947, 26.2009) ccw
  line L4256 (11.5408, 25.882) -> (11.3544, 25.6956)
  arc A4252 (11.3544, 25.6956) -> (11.4622, 25.5878) centre (11.4083, 25.6417) ccw
  line L4257 (11.4622, 25.5878) -> (11.6486, 25.7742)
  arc A4253 (11.6486, 25.7742) -> (11.5408, 25.882) centre (11.5947, 25.8281) ccw
  line L4258 (11.4083, 25.7179) -> (10.6626, 25.7179)
  arc A4254 (10.6626, 25.7179) -> (10.6626, 25.5655) centre (10.6626, 25.6417) ccw
  line L4259 (10.6626, 25.5655) -> (11.4083, 25.5655)
  arc A4255 (11.4083, 25.5655) -> (11.4083, 25.7179) centre (11.4083, 25.6417) ccw
  line L4260 (10.7165, 25.6956) -> (10.5301, 25.882)
  arc A4256 (10.5301, 25.882) -> (10.4223, 25.7742) centre (10.4762, 25.8281) ccw
  line L4261 (10.4223, 25.7742) -> (10.6087, 25.5878)
  arc A4257 (10.6087, 25.5878) -> (10.7165, 25.6956) centre (10.6626, 25.6417) ccw
  line L4262 (10.5524, 25.8281) -> (10.5524, 26.2009)
  arc A4258 (10.5524, 26.2009) -> (10.4, 26.2009) centre (10.4762, 26.2009) ccw
  line L4263 (10.4, 26.2009) -> (10.4, 25.8281)
  arc A4259 (10.4, 25.8281) -> (10.5524, 25.8281) centre (10.4762, 25.8281) ccw
  line L4264 (10.5301, 26.147) -> (10.7165, 26.3335)
  arc A4260 (10.7165, 26.3335) -> (10.6087, 26.4413) centre (10.6626, 26.3874) ccw
  line L4265 (10.6087, 26.4413) -> (10.4223, 26.2548)
  arc A4261 (10.4223, 26.2548) -> (10.5301, 26.147) centre (10.4762, 26.2009) ccw
  line L4266 (10.6626, 26.3112) -> (11.4083, 26.3112)
  arc A4262 (11.4083, 26.3112) -> (11.4083, 26.4636) centre (11.4083, 26.3874) ccw
  line L4267 (11.4083, 26.4636) -> (10.6626, 26.4636)
  arc A4263 (10.6626, 26.4636) -> (10.6626, 26.3112) centre (10.6626, 26.3874) ccw
  line L4268 (11.3544, 26.3335) -> (11.5408, 26.147)
  arc A4264 (11.5408, 26.147) -> (11.6486, 26.2548) centre (11.5947, 26.2009) ccw
  line L4269 (11.6486, 26.2548) -> (11.4622, 26.4413)
  arc A4265 (11.4622, 26.4413) -> (11.3544, 26.3335) centre (11.4083, 26.3874) ccw
  line L4270 (12.5062, 1.3427) -> (13.6247, 1.3427)
  arc A4266 (13.6247, 1.3427) -> (13.6247, 1.4951) centre (13.6247, 1.4189) ccw
  line L4271 (13.6247, 1.4951) -> (12.5062, 1.4951)
  arc A4267 (12.5062, 1.4951) -> (12.5062, 1.3427) centre (12.5062, 1.4189) ccw
  line L4272 (13.667, 1.4823) -> (12.5485, 2.228)
  arc A4268 (12.5485, 2.228) -> (12.4639, 2.1012) centre (12.5062, 2.1646) ccw
  line L4273 (12.4639, 2.1012) -> (13.5824, 1.3555)
  arc A4269 (13.5824, 1.3555) -> (13.667, 1.4823) centre (13.6247, 1.4189) ccw
  line L4274 (12.5062, 2.0884) -> (13.6247, 2.0884)
  arc A4270 (13.6247, 2.0884) -> (13.6247, 2.2408) centre (13.6247, 2.1646) ccw
  line L4275 (13.6247, 2.2408) -> (12.5062, 2.2408)
  arc A4271 (12.5062, 2.2408) -> (12.5062, 2.0884) centre (12.5062, 2.1646) ccw
  line L4276 (13.5485, 3.1474) -> (13.5485, 2.7746)
  arc A4272 (13.5485, 2.7746) -> (13.7009, 2.7746) centre (13.6247, 2.7746) ccw
  line L4277 (13.7009, 2.7746) -> (13.7009, 3.1474)
  arc A4273 (13.7009, 3.1474) -> (13.5485, 3.1474) centre (13.6247, 3.1474) ccw
  line L4278 (13.5708, 2.8285) -> (13.3844, 2.6421)
  arc A4274 (13.3844, 2.6421) -> (13.4922, 2.5343) centre (13.4383, 2.5882) ccw
  line L4279 (13.4922, 2.5343) -> (13.6786, 2.7207)
  arc A4275 (13.6786, 2.7207) -> (13.5708, 2.8285) centre (13.6247, 2.7746) ccw
  line L4280 (13.4383, 2.6644) -> (12.6926, 2.6644)
  arc A4276 (12.6926, 2.6644) -> (12.6926, 2.512) centre (12.6926, 2.5882) ccw
  line L4281 (12.6926, 2.512) -> (13.4383, 2.512)
  arc A4277 (13.4383, 2.512) -> (13.4383, 2.6644) centre (13.4383, 2.5882) ccw
  line L4282 (12.7465, 2.6421) -> (12.5601, 2.8285)
  arc A4278 (12.5601, 2.8285) -> (12.4523, 2.7207) centre (12.5062, 2.7746) ccw
  line L4283 (12.4523, 2.7207) -> (12.6387, 2.5343)
  arc A4279 (12.6387, 2.5343) -> (12.7465, 2.6421) centre (12.6926, 2.5882) ccw
  line L4284 (12.5824, 2.7746) -> (12.5824, 3.1474)
  arc A4280 (12.5824, 3.1474) -> (12.43, 3.1474) centre (12.5062, 3.1474) ccw
  line L4285 (12.43, 3.1474) -> (12.43, 2.7746)
  arc A4281 (12.43, 2.7746) -> (12.5824, 2.7746) centre (12.5062, 2.7746) ccw
  line L4286 (12.5601, 3.0935) -> (12.7465, 3.28)
  arc A4282 (12.7465, 3.28) -> (12.6387, 3.3878) centre (12.6926, 3.3339) ccw
  line L4287 (12.6387, 3.3878) -> (12.4523, 3.2013)
  arc A4283 (12.4523, 3.2013) -> (12.5601, 3.0935) centre (12.5062, 3.1474) ccw
  line L4288 (12.6926, 3.2577) -> (13.4383, 3.2577)
  arc A4284 (13.4383, 3.2577) -> (13.4383, 3.4101) centre (13.4383, 3.3339) ccw
  line L4289 (13.4383, 3.4101) -> (12.6926, 3.4101)
  arc A4285 (12.6926, 3.4101) -> (12.6926, 3.2577) centre (12.6926, 3.3339) ccw
  line L4290 (13.3844, 3.28) -> (13.5708, 3.0935)
  arc A4286 (13.5708, 3.0935) -> (13.6786, 3.2013) centre (13.6247, 3.1474) ccw
  line L4291 (13.6786, 3.2013) -> (13.4922, 3.3878)
  arc A4287 (13.4922, 3.3878) -> (13.3844, 3.28) centre (13.4383, 3.3339) ccw
  line L4292 (13.6247, 3.8337) -> (12.879, 3.8337)
  arc A4288 (12.879, 3.8337) -> (12.879, 3.6813) centre (12.879, 3.7575) ccw
  line L4293 (12.879, 3.6813) -> (13.6247, 3.6813)
  arc A4289 (13.6247, 3.6813) -> (13.6247, 3.8337) centre (13.6247, 3.7575) ccw
  line L4294 (12.9329, 3.8114) -> (12.5601, 4.1842)
  arc A4290 (12.5601, 4.1842) -> (12.4523, 4.0764) centre (12.5062, 4.1303) ccw
  line L4295 (12.4523, 4.0764) -> (12.8251, 3.7036)
  arc A4291 (12.8251, 3.7036) -> (12.9329, 3.8114) centre (12.879, 3.7575) ccw
  line L4296 (12.5601, 4.0764) -> (12.9329, 4.4493)
  arc A4292 (12.9329, 4.4493) -> (12.8251, 4.5571) centre (12.879, 4.5032) ccw
  line L4297 (12.8251, 4.5571) -> (12.4523, 4.1842)
  arc A4293 (12.4523, 4.1842) -> (12.5601, 4.0764) centre (12.5062, 4.1303) ccw
  line L4298 (12.879, 4.427) -> (13.6247, 4.427)
  arc A4294 (13.6247, 4.427) -> (13.6247, 4.5794) centre (13.6247, 4.5032) ccw
  line L4299 (13.6247, 4.5794) -> (12.879, 4.5794)
  arc A4295 (12.879, 4.5794) -> (12.879, 4.427) centre (12.879, 4.5032) ccw
  line L4300 (12.43, 6.8418) -> (12.43, 6.0961)
  arc A4296 (12.43, 6.0961) -> (12.5824, 6.0961) centre (12.5062, 6.0961) ccw
  line L4301 (12.5824, 6.0961) -> (12.5824, 6.8418)
  arc A4297 (12.5824, 6.8418) -> (12.43, 6.8418) centre (12.5062, 6.8418) ccw
  line L4302 (12.5601, 6.0422) -> (13.3058, 6.7879)
  arc A4298 (13.3058, 6.7879) -> (13.198, 6.8957) centre (13.2519, 6.8418) ccw
  line L4303 (13.198, 6.8957) -> (12.4523, 6.15)
  arc A4299 (12.4523, 6.15) -> (12.5601, 6.0422) centre (12.5062, 6.0961) ccw
  line L4304 (13.2519, 6.7656) -> (13.4383, 6.7656)
  arc A4300 (13.4383, 6.7656) -> (13.4383, 6.918) centre (13.4383, 6.8418) ccw
  line L4305 (13.4383, 6.918) -> (13.2519, 6.918)
  arc A4301 (13.2519, 6.918) -> (13.2519, 6.7656) centre (13.2519, 6.8418) ccw
  line L4306 (13.3844, 6.7879) -> (13.5708, 6.6014)
  arc A4302 (13.5708, 6.6014) -> (13.6786, 6.7092) centre (13.6247, 6.6553) ccw
  line L4307 (13.6786, 6.7092) -> (13.4922, 6.8957)
  arc A4303 (13.4922, 6.8957) -> (13.3844, 6.7879) centre (13.4383, 6.8418) ccw
  line L4308 (13.5485, 6.6553) -> (13.5485, 6.2825)
  arc A4304 (13.5485, 6.2825) -> (13.7009, 6.2825) centre (13.6247, 6.2825) ccw
  line L4309 (13.7009, 6.2825) -> (13.7009, 6.6553)
  arc A4305 (13.7009, 6.6553) -> (13.5485, 6.6553) centre (13.6247, 6.6553) ccw
  line L4310 (13.5708, 6.3364) -> (13.3844, 6.15)
  arc A4306 (13.3844, 6.15) -> (13.4922, 6.0422) centre (13.4383, 6.0961) ccw
  line L4311 (13.4922, 6.0422) -> (13.6786, 6.2286)
  arc A4307 (13.6786, 6.2286) -> (13.5708, 6.3364) centre (13.6247, 6.2825) ccw
  line L4312 (12.6926, 7.1892) -> (13.4383, 7.1892)
  arc A4308 (13.4383, 7.1892) -> (13.4383, 7.3416) centre (13.4383, 7.2654) ccw
  line L4313 (13.4383, 7.3416) -> (12.6926, 7.3416)
  arc A4309 (12.6926, 7.3416) -> (12.6926, 7.1892) centre (12.6926, 7.2654) ccw